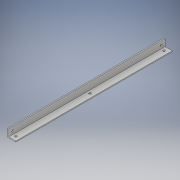
# Autodesk Inventor part: Part2
Saved by Autodesk Inventor 2017 (Build 210142000, 142)
## iProperties
Created: 2018-10-17
Part Number: Part2
Material: Generic
Document SubType Name: Modeling
Designer: ddeboer
Density: 1 g/cm^3
Appearance: Default
Author: ddeboer
Autodesk Inventor part; units mm, degrees
ref_plane "YZ Plane" through (0, 0, 0) normal (1, 0, 0) x (0, 1, 0)
ref_plane "XZ Plane" through (0, 0, 0) normal (0, 1, 0) x (-1, 0, 0)
ref_plane "XY Plane" through (0, 0, 0) normal (0, 0, 1) x (1, 0, 0)
sketch "Sketch1" plane through (0, 0, 0) normal (0, 0, 1) x (1, 0, 0)
  line L0 (0, 25.4) -> (0, 0)
  line L1 (0, 0) -> (25.4, 0)
  line L2 (3.175, 25.4) -> (3.175, 4.953)
  line L3 (4.953, 3.175) -> (25.4, 3.175)
  line L4 (0, 25.4) -> (3.175, 25.4)
  line L5 (25.4, 3.175) -> (25.4, 0)
  line L6 (3.175, 4.953) -> (3.175, 3.175)
  line L7 (4.953, 3.175) -> (3.175, 3.175)
  dimension "d0" = 25.4
  dimension "d1" = 25.4
  dimension "d2" = 3.175
  constraints: 18 end point, 3 perpendicular, 3 vertical, 2 point on line, 1 horizontal, 1 other
  measures "d0" distance of L0.start L0.end
  measures "d1" distance of L0.end L1.end
  measures "d2" distance between parallel lines of L2 L0
extrude "Extrusion1" add sketch "Sketch1" along normal blind 492.125
sketch "Sketch2" plane through (3.175, 3.175, 0) normal (0, 1, 0) x (1, 0, 0)
  circle A0 centre (9.525, -479.425) radius 2.8398
  line L0 (22.225, -492.125) -> (0, -492.125) projected
  line L1 (22.225, 0) -> (22.225, -492.125) projected
  circle A1 centre (9.525, -12.7) radius 2.8398
  line L2 (22.225, 0) -> (0, 0) projected
  point P0 (-3.175, 0)
  point P1 (1.778, -492.125)
  point P2 (1.778, 0)
  dimension "d5" = 12.7
  dimension "d6" = 12.7
  dimension "d9" = 466.725
  dimension "d31" = 12.7
  constraints: 2 centre point, 1 vertical, 2 other
  measures "d5" distance from line of A0.centre L0
  measures "d6" distance from line of A0.centre L1
  measures "d9" distance of A0.centre A1.centre
  measures "d31" distance from line of A1.centre L2
hole "rail" at (12.7, 3.175, 479.425) at (12.7, 3.175, 12.7) direction (0, -1, 0) diameter 6.7564 depth 25.4 tip angle 118 clearance for "Flat Head Machine Screw (82)" size "1/4" standard "Ansi Unified Screw Threads"
sketch "Sketch7" plane through (3.175, 3.175, 0) normal (1, 0, 0) x (0, 0, -1)
  circle A0 centre (-479.425, 9.525) radius 2.8124
  line L0 (0, 22.225) -> (-492.125, 22.225) projected
  line L1 (-492.125, 0) -> (-492.125, 22.225) projected
  circle A1 centre (-12.7, 9.525) radius 2.8124
  point P0 (0, -3.175)
  dimension "d43" = 12.7
  dimension "d44" = 12.7
  dimension "d47" = 466.725
  constraints: 2 centre point, 1 horizontal, 2 other
  measures "d43" distance from line of A0.centre L0
  measures "d44" distance from line of A0.centre L1
  measures "d47" distance of A0.centre A1.centre
hole "mount" at (3.175, 12.7, 479.425) at (3.175, 12.7, 12.7) direction (-1, 0, 0) diameter 6.7564 depth 25.4 tip angle 118 clearance for "Flat Head Machine Screw (82)" size "1/4" standard "Ansi Unified Screw Threads"
sketch "Sketch8" plane through (3.175, 3.175, 0) normal (0, 1, 0) x (1, 0, 0)
  circle A0 centre (9.525, -479.425) radius 3.3782 projected
  circle A1 centre (9.525, -12.7) radius 3.3782 projected
  line L0 (9.525, -479.425) -> (9.525, -12.7) construction
  circle A2 centre (9.525, -246.0625) radius 3.3782
  point P0 (-3.175, 0)
  constraints: 2 end point, 1 centre point, 1 midpoint, 1 vertical
hole "Hole5" at (12.7, 3.175, 246.0625) direction (0, -1, 0) diameter 6.7564 depth 25.4 tip angle 118 clearance for "Flat Head Machine Screw (82)" size "1/4" standard "Ansi Unified Screw Threads"
body "Solid1"
